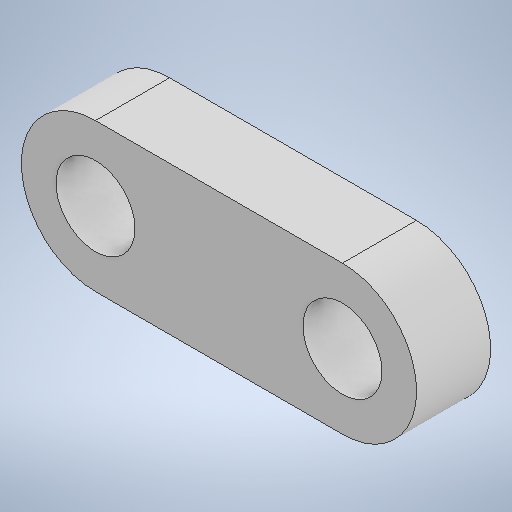
# Autodesk Inventor part: Wires Input Orientation
Saved by Autodesk Inventor 2025.4 (Build 294407000, 407)
## iProperties
Created: 2026-05-09
Part Number: Wires Input Orientation
Material: Generic
Document SubType Name: Sheet Metal
Designer: lenovo
Density: 1 g/cm^3
Sheet Metal Rule: Default_mm
Appearance: Default
Author: lenovo
Autodesk Inventor part; units mm, degrees
ref_plane "YZ Plane" through (0, 0, 0) normal (1, 0, 0) x (0, 1, 0)
ref_plane "XZ Plane" through (0, 0, 0) normal (0, 1, 0) x (-1, 0, 0)
ref_plane "XY Plane" through (0, 0, 0) normal (0, 0, 1) x (1, 0, 0)
sketch "Sketch1" plane through (0, 0, 0) normal (0, 0, 1) x (1, 0, 0)
  line L0 (-5, 0) -> (5, 0) construction
  line L1 (-5, -3) -> (5, -3)
  line L2 (5, 3) -> (-5, 3)
  arc A0 (-5, 3) -> (-5, -3) centre (-5, 0) ccw
  arc A1 (5, -3) -> (5, 3) centre (5, 0) ccw
  circle A2 centre (5, 0) radius 1.6
  circle A3 centre (-5, 0) radius 1.6
  point P0 (0, 0)
  dimension "d0" = 3
  dimension "d1" = 10
  dimension "d2" = 3.2
  dimension "d3" = 3.2
  measures "d0" radius of A1
  measures "d1" distance of L0.start L0.end
  measures "d2" diameter of A2
  measures "d3" diameter of A3
extrude "Plate1" add sketch "Sketch1" along normal blind 3
equation "\"d4\" = Thickness"
equation "\"BendRadius\" = Thickness"
equation "\"BendReliefWidth\" = Thickness"
equation "\"BendReliefDepth\" = 0.5 * Thickness"
equation "\"CornerReliefSize\" = 4 * Thickness"
equation "\"MinimumRemnant\" = 2 * Thickness"
equation "\"TransitionRadius\" = BendRadius"
equation "\"JacobiRadiusSize\" = BendRadius"
equation "\"GapSize\" = Thickness"
equation "\"Thickness\" = 3"
body "Solid1"
